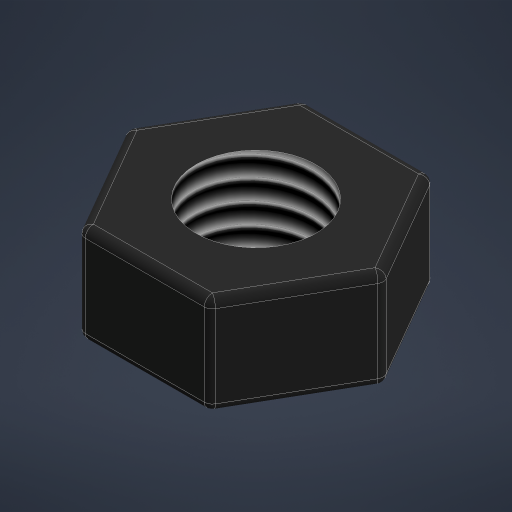
# Autodesk Inventor part: M3 Nut
Saved by Autodesk Inventor 2024 (Build 280153000, 153)
## iProperties
Created: 2024-10-26
Part Number: M3 Nut
Material: Generic
Document SubType Name: Modeling
Designer: jerem
Density: 1 g/cm^3
Appearance: Default
Author: jerem
Autodesk Inventor part; units mm, degrees
ref_plane "YZ Plane" through (0, 0, 0) normal (1, 0, 0) x (0, 1, 0)
ref_plane "XZ Plane" through (0, 0, 0) normal (0, 1, 0) x (-1, 0, 0)
ref_plane "XY Plane" through (0, 0, 0) normal (0, 0, 1) x (1, 0, 0)
sketch "Sketch1" plane through (0, 0, 0) normal (0, 1, 0) x (-1, 0, 0)
  line L0 (3.1466, 0) -> (1.5733, -2.725)
  line L1 (1.5733, -2.725) -> (-1.5733, -2.725)
  line L2 (-1.5733, -2.725) -> (-3.1466, 0)
  line L3 (-3.1466, 0) -> (-1.5733, 2.725)
  line L4 (-1.5733, 2.725) -> (1.5733, 2.725)
  line L5 (1.5733, 2.725) -> (3.1466, 0)
  circle A0 centre (0, 0) radius 1.465
  dimension "d0" = 5.45
  dimension "d1" = 2.93
  constraints: 12 end point, 2 coincident, 1 centre point, 1 horizontal, 13 other
  measures "d0" distance between parallel lines of L4 L1
  measures "d1" diameter of A0
extrude "Extrusion1" add sketch "Sketch1" along normal blind 2.42
fillet "Fillet1" radius 0.2 18 edges at (2.3599, 2.42, 1.3625) (0, 2.42, 2.725) (1.5733, 1.21, 2.725) (0, 0, 2.725) (-1.5733, 1.21, 2.725) (2.3599, 0, 1.3625) (3.1466, 1.21, 0) (1.5733, 1.21, -2.725) (2.3599, 2.42, -1.3625) (2.3599, 0, -1.3625) (-1.5733, 1.21, -2.725) (0, 2.42, -2.725) (0, 0, -2.725) (-2.3599, 2.42, 1.3625) (-2.3599, 2.42, -1.3625) (-3.1466, 1.21, 0) (-2.3599, 0, -1.3625) (-2.3599, 0, 1.3625)
thread "Thread1" size "M3x0.5" class "6H" standard "ANSI Metric M Profile" full length
body "Solid1"
